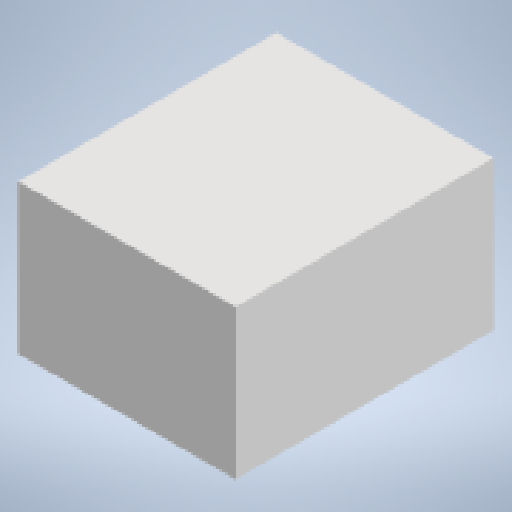
# Autodesk Inventor part: MotorPart1
Saved by Autodesk Inventor 2024 (Build 280153000, 153)
## iProperties
Created: 2024-10-17
Part Number: MotorPart1
Material: 一般
Document SubType Name: Modeling
Designer: jerry
Density: 1 g/cm^3
Appearance: 預設
Author: jerry
Autodesk Inventor part; units mm, degrees
ref_plane "YZ Plane" through (0, 0, 0) normal (1, 0, 0) x (0, 1, 0)
ref_plane "XZ Plane" through (0, 0, 0) normal (0, 1, 0) x (-1, 0, 0)
ref_plane "XY Plane" through (0, 0, 0) normal (0, 0, 1) x (1, 0, 0)
sketch "草圖1" plane through (0, 0, 0) normal (0, 0, 1) x (1, 0, 0)
  line L0 (-40, 27.5) -> (40, 27.5)
  line L1 (40, 27.5) -> (40, -27.5)
  line L2 (40, -27.5) -> (-40, -27.5)
  line L3 (-40, -27.5) -> (-40, 27.5)
  line L4 (-40, 27.5) -> (40, -27.5) construction
  line L5 (40, 27.5) -> (-40, -27.5) construction
  circle A0 centre (0, 0) radius 18.5
  circle A1 centre (0, -18.5) radius 30
  circle A2 centre (-30, -18.5) radius 3
  circle A3 centre (30, -18.5) radius 3
  circle A4 centre (0, 18.5) radius 30
  circle A5 centre (-30, 18.5) radius 3
  circle A6 centre (30, 18.5) radius 3
  dimension "d0" = 80
  dimension "d1" = 55
  dimension "d4" = 37
  dimension "d5" = 60
  dimension "d6" = 6
  dimension "d7" = 6
  dimension "d8" = 60
  dimension "d9" = 6
  dimension "d10" = 6
  constraints: 12 end point, 7 centre point, 6 point on circle, 2 midpoint, 2 parallel, 1 coincident, 1 horizontal, 1 perpendicular
  measures "d0" distance of L1.end L2.end
  measures "d1" distance of L0.end L1.end
  measures "d4" diameter of A0
  measures "d5" diameter of A1
  measures "d6" diameter of A2
  measures "d7" diameter of A3
  measures "d8" diameter of A4
  measures "d9" diameter of A5
  measures "d10" diameter of A6
extrude "擠出1" add sketch "草圖1" along normal blind 95 contours L0 A4 A5 A1 A2 L2 L3 | L0 A4 A6 A1 A0 A5 | L0 L1 L2 A1 A3 A4 A6 | A1 A2 A4 A0 A3 L2 | A1 A0 A4 | A4 A0 A1 | A1 A0 A4 | A0 A1 | A4 A0
sketch "草圖2" plane through (-40, -27.5, 0) normal (-1, 0, 0) x (0, 0, 1)
  line L0 (95, 0) -> (95, 55) projected
  circle A0 centre (95, 0) radius 27.5
  circle A1 centre (95, 27.5) radius 23
  circle A2 centre (72, 27.5) radius 15
  point P0 (0, 27.5)
  dimension "d11" = 46
  dimension "d12" = 30
  constraints: 1 centre point, 1 horizontal alignment, 1 midpoint, 1 vertical alignment, 4 other
  measures "d12" diameter of A2
extrude "擠出2" cut sketch "草圖2" along normal through all both and the other way through all contours A2 A0 A1 | A1 A0 A2 | A0 A1 A2 | A0 A2 A1 picked at (73.0639, 14.4683) picked at (77.5879, 17.5315) picked at (79.9817, 30.5353) picked at (67.7059, 31.4722)
sketch "草圖3" plane through (-40, 27.5, 0) normal (0, 1, 0) x (1, 0, 0)
  circle A0 centre (40, 0) radius 40
  circle A1 centre (40, -40) radius 15
  dimension "d15" = 80
  dimension "d16" = 30
  constraints: 1 centre point, 1 coincident, 1 vertical alignment, 2 other
  measures "d16" diameter of A1
extrude "擠出3" add sketch "草圖3" along normal blind 5 and the other way blind 60 contours A1 A0 | A0 A1 picked at (35.277, -35.2849) picked at (34.8016, -43.9729)
